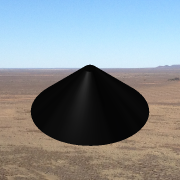
# Autodesk Inventor part: splash-top
Saved by Autodesk Inventor 2013 SP2 (Build 170200200, 200)
## iProperties
Company: HERA Project
Created: 2013-05-31
Part Number: splash-top
Material: Acetal Resin, Black
Document SubType Name: Modeling
Designer: David DeBoer
Density: 1.425 g/cm^3
Description: Splash top piece (absorber)
Mass: 1072.45 g
Surface Area: 1266.96 cm^2
Volume: 752.599 cm^3
Author: David DeBoer
Title: Splash
Autodesk Inventor part; units mm, degrees
ref_plane "YZ Plane" through (0, 0, 0) normal (1, 0, 0) x (0, 1, 0)
ref_plane "XZ Plane" through (0, 0, 0) normal (0, 1, 0) x (-1, 0, 0)
ref_plane "XY Plane" through (0, 0, 0) normal (0, 0, 1) x (1, 0, 0)
sketch "Sketch6" plane through (0, 0, 0) normal (0, 0, 1) x (1, 0, 0)
  line L0 (-121.9668, 335.4799) -> (0, 457.4895)
  line L1 (-102.8093, 335.4799) -> (0, 438.3253)
  line L2 (0, 457.4895) -> (0, 438.3253)
  line L3 (0, -91.4979) -> (0, 548.9874) projected
  line L4 (-121.9668, 335.4799) -> (-102.8093, 335.4799)
  point P0 (0, 0)
  constraints: 8 end point, 1 parallel, 1 perpendicular, 1 vertical
revolve "Revolution2" add sketch "Sketch6" angle 360 about axis through (0, -10, 0) along (0, 1, 0)
sketch "Sketch7" plane through (0, 0, 0) normal (0, 1, 0) x (-1, 0, 0)
  circle A0 centre (0, 0) radius 12.7
  dimension "d12" = 25.4
  constraints: 1 centre point, 1 coincident
  measures "d12" diameter of A0
extrude "Extrusion3" cut sketch "Sketch7" along normal blind 762
body "Solid1"
